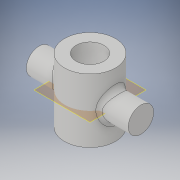
# Autodesk Inventor part: holder
Saved by Autodesk Inventor 2019 (Build 230136000, 136)
## iProperties
Created: 2021-05-24
Part Number: holder
Material: Genérico
Document SubType Name: Modeling
Designer: Juan M. Casillas
Density: 1 g/cm^3
Appearance: Valor por defecto
Author: Juan M. Casillas
## iProperties of the stored document holder_3DPrint.ipt
Created: 2021-05-24
Part Number: holder_3DPrint
Material: Genérico
Document SubType Name: Modeling
Designer: Juan M. Casillas
Density: 1 g/cm^3
Appearance: Valor por defecto
Author: Juan M. Casillas
Autodesk Inventor part; units mm, degrees
ref_plane "YZ Plane" through (0, 0, 0) normal (1, 0, 0) x (0, 1, 0)
ref_plane "XZ Plane" through (0, 0, 0) normal (0, 1, 0) x (-1, 0, 0)
ref_plane "XY Plane" through (0, 0, 0) normal (0, 0, 1) x (1, 0, 0)
sketch "Sketch1" plane through (0, 0, 0) normal (0, 1, 0) x (-1, 0, 0)
  circle A0 centre (0, 0) radius 5.45
  circle A1 centre (0, 0) radius 10
  dimension "d0" = 10.9
  dimension "d1" = 20
  constraints: 2 centre point, 2 coincident
  measures "d0" diameter of A0
  measures "d1" diameter of A1
extrude "Extrusion1" add sketch "Sketch1" along normal blind 25
ref_plane "Work Plane1" through (0, 12.5, 0) normal (0, 1, 0) x (1, 0, 0)
sketch "Sketch2" plane through (0, 0, 0) normal (1, 0, 0) x (0, 1, 0)
  line L0 (25, -10) -> (25, 10) construction
  line L1 (0, 10) -> (0, -10) construction
  circle A0 centre (12.4366, 0) radius 5
  point P0 (0, 0)
  dimension "d4" = 10
  constraints: 1 centre point
  measures "d4" diameter of A0
extrude "Extrusion2" add sketch "Sketch2" along normal blind 20 and the other way blind 20
sketch "Sketch3" plane through (0, 25, 0) normal (0, 1, 0) x (1, 0, 0)
  circle A0 centre (0, 0) radius 5.45 projected
extrude "Extrusion3" cut sketch "Sketch3" against normal through all
fillet "Fillet1" radius 2 3 edges at (-8.6603, 12.431, 5) (-8.6603, 12.4422, -5) (10, 7.4366, 0.0174)
body "Solid1"
